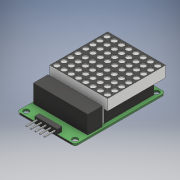
# Autodesk Inventor part: learnbotMatrizLed
Saved by Autodesk Inventor 2017 (Build 210142000, 142)
## iProperties
Part Number: learnbotMatrizLed
Material: Genérico
Document SubType Name: Modeling
Designer: rober
Density: 1 g/cm^3
Appearance: Valor por defecto
Author: rober
Autodesk Inventor part; units mm, degrees
ref_plane "YZ Plane" through (0, 0, 0) normal (1, 0, 0) x (0, 1, 0)
ref_plane "XZ Plane" through (0, 0, 0) normal (0, 1, 0) x (-1, 0, 0)
ref_plane "XY Plane" through (0, 0, 0) normal (0, 0, 1) x (1, 0, 0)
sketch "Boceto1" plane through (0, 0, 0) normal (0, 0, 1) x (1, 0, 0)
  line L0 (-0.15, 0.15) -> (-0.15, 4.85)
  line L1 (0, 5) -> (2.9, 5)
  line L2 (3.05, 4.85) -> (3.05, 0.15)
  line L3 (2.9, 0) -> (0, 0)
  arc A0 (2.9, 0) -> (3.05, 0.15) centre (2.9, 0.15) ccw
  arc A1 (-0.15, 0.15) -> (0, 0) centre (0, 0.15) ccw
  line L4 (3.05, 1.6) -> (3.05, 0.8)
  circle A2 centre (0.1, 0.25) radius 0.15
  circle A3 centre (2.8, 0.25) radius 0.15
  line L5 (0.925, 0) -> (0.925, -0.6)
  line L6 (0.975, 0) -> (0.975, -0.6)
  line L7 (0.925, -0.6) -> (0.975, -0.6)
  line L8 (1.175, 0) -> (1.175, -0.6)
  line L9 (1.225, 0) -> (1.225, -0.6)
  line L10 (1.175, -0.6) -> (1.225, -0.6)
  line L11 (1.425, 0) -> (1.425, -0.6)
  line L12 (1.475, 0) -> (1.475, -0.6)
  line L13 (1.425, -0.6) -> (1.475, -0.6)
  line L14 (1.675, 0) -> (1.675, -0.6)
  line L15 (1.725, 0) -> (1.725, -0.6)
  line L16 (1.675, -0.6) -> (1.725, -0.6)
  line L17 (1.925, 0) -> (1.925, -0.6)
  line L18 (1.975, 0) -> (1.975, -0.6)
  line L19 (1.925, -0.6) -> (1.975, -0.6)
  line L20 (0.925, 5) -> (0.925, 5.45)
  line L21 (0.975, 5) -> (0.975, 5.45)
  line L22 (0.925, 5.45) -> (0.975, 5.45)
  line L23 (1.175, 5) -> (1.175, 5.45)
  line L24 (1.225, 5) -> (1.225, 5.45)
  line L25 (1.175, 5.45) -> (1.225, 5.45)
  line L26 (1.425, 5) -> (1.425, 5.45)
  line L27 (1.475, 5) -> (1.475, 5.45)
  line L28 (1.425, 5.45) -> (1.475, 5.45)
  line L29 (1.675, 5) -> (1.675, 5.45)
  line L30 (1.725, 5) -> (1.725, 5.45)
  line L31 (1.675, 5.45) -> (1.725, 5.45)
  line L32 (1.925, 5) -> (1.925, 5.45)
  line L33 (1.975, 5) -> (1.975, 5.45)
  line L34 (1.925, 5.45) -> (1.975, 5.45)
  arc A4 (3.05, 4.85) -> (2.9, 5) centre (2.9, 4.85) ccw
  arc A5 (0, 5) -> (-0.15, 4.85) centre (0, 4.85) ccw
  circle A6 centre (0.1, 4.75) radius 0.15
  circle A7 centre (2.8, 4.75) radius 0.15
  constraints: 66 end point, 8 centre point, 8 point on circle, 2 point on line, 26 other
extrude "Extrusión1" add sketch "Boceto1" against normal blind 0.1 contours L0 A5 L1 A4 L2 A0 L3 A1
sketch "Boceto2" plane through (-0.15, 0.15, 0) normal (-1, 0, 0) x (0, 0, 1)
  line L0 (0.7, 4.85) -> (1.3, 4.85)
  line L1 (1.3, 4.85) -> (1.3, 1.65)
  line L2 (-0.1, 4.85) -> (-0.1, -0.15)
  line L3 (0, 1.65) -> (1.3, 1.65)
  line L4 (0, 1.45) -> (1, 1.45)
  line L5 (1, 1.45) -> (1, 0.65)
  line L6 (1, 0.65) -> (0, 0.65)
  line L7 (-0.1, -0.15) -> (0, -0.15)
  line L8 (0, -0.15) -> (0, 4.85)
  line L9 (0, 0.1) -> (0.25, 0.1)
  line L10 (0.25, 0.1) -> (0.25, -0.15)
  line L11 (0.25, -0.15) -> (0, -0.15)
  line L12 (0.1, -0.75) -> (0.15, -0.75)
  line L13 (0.15, -0.75) -> (0.15, -0.15)
  line L14 (0.1, -0.15) -> (0.1, -0.75)
  line L15 (0.1, 5.3) -> (0.15, 5.3)
  line L16 (0.15, 5.3) -> (0.15, 4.7)
  line L17 (0.1, 4.7) -> (0.1, 5.3)
  line L18 (1.3, 4.85) -> (0.7, 4.85)
  line L19 (0.7, 4.85) -> (0.7, 1.65)
  line L20 (0, 4.7) -> (0.7, 4.7)
  line L21 (0, 4.85) -> (-0.1, 4.85)
  constraints: 44 end point, 11 point on line
extrude "Extrusión2" add sketch "Boceto2" against normal blind 3.2 contours L0 L1 L3 L19 | L19 L3 L8 L20 | L4 L5 L6 L8
sketch "Boceto3" plane through (-0.15, 1.8, 1.3) normal (0, 0, 1) x (1, 0, 0)
  line L0 (0, -1.65) -> (0, 3.2)
  line L1 (0, 3.2) -> (3.2, 3.2)
  line L2 (3.2, 3.2) -> (3.2, -1.65)
  line L3 (3.05, -1.8) -> (0.15, -1.8)
  line L4 (3.2, 0) -> (0, 0)
  line L5 (3.2, -0.2) -> (3.2, -1)
  line L6 (3.2, -1) -> (0, -1)
  line L7 (3.2, -0.2) -> (0, -0.2)
  circle A0 centre (0.25, -1.55) radius 0.15
  circle A1 centre (2.95, -1.55) radius 0.15
  arc A2 (0, -1.65) -> (0.15, -1.8) centre (0.15, -1.65) ccw
  arc A3 (3.05, -1.8) -> (3.2, -1.65) centre (3.05, -1.65) ccw
  circle A4 centre (0.2, 0.1969) radius 0.15
  circle A5 centre (0.2, 0.5906) radius 0.15
  circle A6 centre (0.2, 0.9719) radius 0.15
  circle A7 centre (0.2, 1.3656) radius 0.15
  circle A8 centre (0.2, 1.7969) radius 0.15
  circle A9 centre (0.2, 2.1906) radius 0.15
  circle A10 centre (0.2, 2.5719) radius 0.15
  circle A11 centre (0.2, 2.9656) radius 0.15
  circle A12 centre (0.6, 0.1969) radius 0.15
  circle A13 centre (0.6, 0.5906) radius 0.15
  circle A14 centre (0.6, 0.9719) radius 0.15
  circle A15 centre (0.6, 1.3656) radius 0.15
  circle A16 centre (0.6, 1.7969) radius 0.15
  circle A17 centre (0.6, 2.1906) radius 0.15
  circle A18 centre (0.6, 2.5719) radius 0.15
  circle A19 centre (0.6, 2.9656) radius 0.15
  circle A20 centre (1, 0.1969) radius 0.15
  circle A21 centre (1, 0.5906) radius 0.15
  circle A22 centre (1, 0.9719) radius 0.15
  circle A23 centre (1, 1.3656) radius 0.15
  circle A24 centre (1, 1.7969) radius 0.15
  circle A25 centre (1, 2.1906) radius 0.15
  circle A26 centre (1, 2.5719) radius 0.15
  circle A27 centre (1, 2.9656) radius 0.15
  circle A28 centre (1.4, 0.1969) radius 0.15
  circle A29 centre (1.4, 0.5906) radius 0.15
  circle A30 centre (1.4, 0.9719) radius 0.15
  circle A31 centre (1.4, 1.3656) radius 0.15
  circle A32 centre (1.4, 1.7969) radius 0.15
  circle A33 centre (1.4, 2.1906) radius 0.15
  circle A34 centre (1.4, 2.5719) radius 0.15
  circle A35 centre (1.4, 2.9656) radius 0.15
  circle A36 centre (1.8, 0.1969) radius 0.15
  circle A37 centre (1.8, 0.5906) radius 0.15
  circle A38 centre (1.8, 0.9719) radius 0.15
  circle A39 centre (1.8, 1.3656) radius 0.15
  circle A40 centre (1.8, 1.7969) radius 0.15
  circle A41 centre (1.8, 2.1906) radius 0.15
  circle A42 centre (1.8, 2.5719) radius 0.15
  circle A43 centre (1.8, 2.9656) radius 0.15
  circle A44 centre (2.2, 0.1969) radius 0.15
  circle A45 centre (2.2, 0.5906) radius 0.15
  circle A46 centre (2.2, 0.9719) radius 0.15
  circle A47 centre (2.2, 1.3656) radius 0.15
  circle A48 centre (2.2, 1.7969) radius 0.15
  circle A49 centre (2.2, 2.1906) radius 0.15
  circle A50 centre (2.2, 2.5719) radius 0.15
  circle A51 centre (2.2, 2.9656) radius 0.15
  circle A52 centre (2.6, 0.1969) radius 0.15
  circle A53 centre (2.6, 0.5906) radius 0.15
  circle A54 centre (2.6, 0.9719) radius 0.15
  circle A55 centre (2.6, 1.3656) radius 0.15
  circle A56 centre (2.6, 1.7969) radius 0.15
  circle A57 centre (2.6, 2.1906) radius 0.15
  circle A58 centre (2.6, 2.5719) radius 0.15
  circle A59 centre (2.6, 2.9656) radius 0.15
  circle A60 centre (3, 0.1969) radius 0.15
  circle A61 centre (3, 0.5906) radius 0.15
  circle A62 centre (3, 0.9719) radius 0.15
  circle A63 centre (3, 1.3656) radius 0.15
  circle A64 centre (3, 1.7969) radius 0.15
  circle A65 centre (3, 2.1906) radius 0.15
  circle A66 centre (3, 2.5719) radius 0.15
  circle A67 centre (3, 2.9656) radius 0.15
  line L8 (0.975, -1.8) -> (0.975, -1.55)
  line L9 (0.975, -1.55) -> (2.225, -1.55)
  line L10 (2.225, -1.55) -> (2.225, -1.8)
  line L11 (1.225, -1.8) -> (1.225, -1.55)
  line L12 (1.475, -1.8) -> (1.475, -1.55)
  line L13 (1.725, -1.8) -> (1.725, -1.55)
  line L14 (1.975, -1.8) -> (1.975, -1.55)
  line L15 (1.075, -1.8) -> (1.075, -2.4)
  line L16 (1.125, -1.8) -> (1.125, -2.4)
  line L17 (1.075, -2.4) -> (1.125, -2.4)
  line L18 (1.325, -1.8) -> (1.325, -2.4)
  line L19 (1.375, -1.8) -> (1.375, -2.4)
  line L20 (1.325, -2.4) -> (1.375, -2.4)
  line L21 (1.575, -1.8) -> (1.575, -2.4)
  line L22 (1.625, -1.8) -> (1.625, -2.4)
  line L23 (1.575, -2.4) -> (1.625, -2.4)
  line L24 (1.825, -1.8) -> (1.825, -2.4)
  line L25 (1.875, -1.8) -> (1.875, -2.4)
  line L26 (1.825, -2.4) -> (1.875, -2.4)
  line L27 (2.075, -1.8) -> (2.075, -2.4)
  line L28 (2.125, -1.8) -> (2.125, -2.4)
  line L29 (2.075, -2.4) -> (2.125, -2.4)
  line L30 (1.075, 3.2) -> (1.075, 3.65)
  line L31 (1.125, 3.2) -> (1.125, 3.65)
  line L32 (1.075, 3.65) -> (1.125, 3.65)
  line L33 (1.325, 3.2) -> (1.325, 3.65)
  line L34 (1.375, 3.2) -> (1.375, 3.65)
  line L35 (1.325, 3.65) -> (1.375, 3.65)
  line L36 (1.575, 3.2) -> (1.575, 3.65)
  line L37 (1.625, 3.2) -> (1.625, 3.65)
  line L38 (1.575, 3.65) -> (1.625, 3.65)
  line L39 (1.825, 3.2) -> (1.825, 3.65)
  line L40 (1.875, 3.2) -> (1.875, 3.65)
  line L41 (1.825, 3.65) -> (1.875, 3.65)
  line L42 (2.075, 3.2) -> (2.075, 3.65)
  line L43 (2.125, 3.2) -> (2.125, 3.65)
  line L44 (2.075, 3.65) -> (2.125, 3.65)
  line L45 (0, 0) -> (0, 3.2) projected
  line L46 (0, 0) -> (3.2, 0) projected
  line L47 (3.2, 3.2) -> (3.2, 0) projected
  line L48 (0, 3.2) -> (3.2, 3.2) projected
  point P0 (0.15, -1.8)
  constraints: 86 end point, 68 centre point, 10 point on line, 4 point on circle, 32 other
extrude "Extrusión3" cut sketch "Boceto3" against normal blind 0.05 contours A4 | A5 | A6 | A7 | A8 | A9 | A10 | A11 | A12 | A13 | A14 | A15 | A16 | A17 | A18 | A19 | A20 | A21 | A22 | A23 | A24 | A25 | A26 | A27 | A28 | A29 | A30 | A31 | A32 | A33 | A34 | A35 | A36 | A37 | A38 | A39 | A40 | A41 | A42 | A43 | A44 | A45 | A46 | A47 | A48 | A49 | A50 | A51 | A52 | A53 | A54 | A55 | A56 | A57 | A58 | A59 | A60 | A61 | A62 | A63 | A64 | A65 | A66 | A67
sketch "Boceto4" plane through (0, 0, 0) normal (0, 0, 1) x (1, 0, 0)
  line L0 (-0.15, 0.15) -> (-0.15, 5)
  line L1 (-0.15, 5) -> (3.05, 5)
  line L2 (3.05, 5) -> (3.05, 0.15)
  line L3 (2.9, 0) -> (0, 0)
  line L4 (3.05, 1.8) -> (-0.15, 1.8)
  line L5 (3.05, 1.6) -> (3.05, 0.8)
  line L6 (3.05, 0.8) -> (-0.15, 0.8)
  line L7 (3.05, 1.6) -> (-0.15, 1.6)
  circle A0 centre (0.1, 0.25) radius 0.15
  circle A1 centre (2.8, 0.25) radius 0.15
  arc A2 (-0.15, 0.15) -> (0, 0) centre (0, 0.15) ccw
  arc A3 (2.9, 0) -> (3.05, 0.15) centre (2.9, 0.15) ccw
  circle A4 centre (0.05, 1.9969) radius 0.15
  circle A5 centre (0.05, 2.3906) radius 0.15
  circle A6 centre (0.05, 2.7719) radius 0.15
  circle A7 centre (0.05, 3.1656) radius 0.15
  circle A8 centre (0.05, 3.5969) radius 0.15
  circle A9 centre (0.05, 3.9906) radius 0.15
  circle A10 centre (0.05, 4.3719) radius 0.15
  circle A11 centre (0.05, 4.7656) radius 0.15
  circle A12 centre (0.45, 1.9969) radius 0.15
  circle A13 centre (0.45, 2.3906) radius 0.15
  circle A14 centre (0.45, 2.7719) radius 0.15
  circle A15 centre (0.45, 3.1656) radius 0.15
  circle A16 centre (0.45, 3.5969) radius 0.15
  circle A17 centre (0.45, 3.9906) radius 0.15
  circle A18 centre (0.45, 4.3719) radius 0.15
  circle A19 centre (0.45, 4.7656) radius 0.15
  circle A20 centre (0.85, 1.9969) radius 0.15
  circle A21 centre (0.85, 2.3906) radius 0.15
  circle A22 centre (0.85, 2.7719) radius 0.15
  circle A23 centre (0.85, 3.1656) radius 0.15
  circle A24 centre (0.85, 3.5969) radius 0.15
  circle A25 centre (0.85, 3.9906) radius 0.15
  circle A26 centre (0.85, 4.3719) radius 0.15
  circle A27 centre (0.85, 4.7656) radius 0.15
  circle A28 centre (1.25, 1.9969) radius 0.15
  circle A29 centre (1.25, 2.3906) radius 0.15
  circle A30 centre (1.25, 2.7719) radius 0.15
  circle A31 centre (1.25, 3.1656) radius 0.15
  circle A32 centre (1.25, 3.5969) radius 0.15
  circle A33 centre (1.25, 3.9906) radius 0.15
  circle A34 centre (1.25, 4.3719) radius 0.15
  circle A35 centre (1.25, 4.7656) radius 0.15
  circle A36 centre (1.65, 1.9969) radius 0.15
  circle A37 centre (1.65, 2.3906) radius 0.15
  circle A38 centre (1.65, 2.7719) radius 0.15
  circle A39 centre (1.65, 3.1656) radius 0.15
  circle A40 centre (1.65, 3.5969) radius 0.15
  circle A41 centre (1.65, 3.9906) radius 0.15
  circle A42 centre (1.65, 4.3719) radius 0.15
  circle A43 centre (1.65, 4.7656) radius 0.15
  circle A44 centre (2.05, 1.9969) radius 0.15
  circle A45 centre (2.05, 2.3906) radius 0.15
  circle A46 centre (2.05, 2.7719) radius 0.15
  circle A47 centre (2.05, 3.1656) radius 0.15
  circle A48 centre (2.05, 3.5969) radius 0.15
  circle A49 centre (2.05, 3.9906) radius 0.15
  circle A50 centre (2.05, 4.3719) radius 0.15
  circle A51 centre (2.05, 4.7656) radius 0.15
  circle A52 centre (2.45, 1.9969) radius 0.15
  circle A53 centre (2.45, 2.3906) radius 0.15
  circle A54 centre (2.45, 2.7719) radius 0.15
  circle A55 centre (2.45, 3.1656) radius 0.15
  circle A56 centre (2.45, 3.5969) radius 0.15
  circle A57 centre (2.45, 3.9906) radius 0.15
  circle A58 centre (2.45, 4.3719) radius 0.15
  circle A59 centre (2.45, 4.7656) radius 0.15
  circle A60 centre (2.85, 1.9969) radius 0.15
  circle A61 centre (2.85, 2.3906) radius 0.15
  circle A62 centre (2.85, 2.7719) radius 0.15
  circle A63 centre (2.85, 3.1656) radius 0.15
  circle A64 centre (2.85, 3.5969) radius 0.15
  circle A65 centre (2.85, 3.9906) radius 0.15
  circle A66 centre (2.85, 4.3719) radius 0.15
  circle A67 centre (2.85, 4.7656) radius 0.15
  line L8 (0.825, 0) -> (0.825, 0.25)
  line L9 (0.825, 0.25) -> (2.075, 0.25)
  line L10 (2.075, 0.25) -> (2.075, 0)
  line L11 (1.075, 0) -> (1.075, 0.25)
  line L12 (1.325, 0) -> (1.325, 0.25)
  line L13 (1.575, 0) -> (1.575, 0.25)
  line L14 (1.825, 0) -> (1.825, 0.25)
  line L15 (0.925, 0) -> (0.925, -0.6)
  line L16 (0.975, 0) -> (0.975, -0.6)
  line L17 (0.925, -0.6) -> (0.975, -0.6)
  line L18 (1.175, 0) -> (1.175, -0.6)
  line L19 (1.225, 0) -> (1.225, -0.6)
  line L20 (1.175, -0.6) -> (1.225, -0.6)
  line L21 (1.425, 0) -> (1.425, -0.6)
  line L22 (1.475, 0) -> (1.475, -0.6)
  line L23 (1.425, -0.6) -> (1.475, -0.6)
  line L24 (1.675, 0) -> (1.675, -0.6)
  line L25 (1.725, 0) -> (1.725, -0.6)
  line L26 (1.675, -0.6) -> (1.725, -0.6)
  line L27 (1.925, 0) -> (1.925, -0.6)
  line L28 (1.975, 0) -> (1.975, -0.6)
  line L29 (1.925, -0.6) -> (1.975, -0.6)
  line L30 (0.925, 5) -> (0.925, 5.45)
  line L31 (0.975, 5) -> (0.975, 5.45)
  line L32 (0.925, 5.45) -> (0.975, 5.45)
  line L33 (1.175, 5) -> (1.175, 5.45)
  line L34 (1.225, 5) -> (1.225, 5.45)
  line L35 (1.175, 5.45) -> (1.225, 5.45)
  line L36 (1.425, 5) -> (1.425, 5.45)
  line L37 (1.475, 5) -> (1.475, 5.45)
  line L38 (1.425, 5.45) -> (1.475, 5.45)
  line L39 (1.675, 5) -> (1.675, 5.45)
  line L40 (1.725, 5) -> (1.725, 5.45)
  line L41 (1.675, 5.45) -> (1.725, 5.45)
  line L42 (1.925, 5) -> (1.925, 5.45)
  line L43 (1.975, 5) -> (1.975, 5.45)
  line L44 (1.925, 5.45) -> (1.975, 5.45)
  circle A68 centre (0.1, 0.25) radius 0.15 projected
  point P0 (0, 0)
  constraints: 86 end point, 68 centre point, 10 point on line, 4 point on circle, 32 other
extrude "Extrusión4" add sketch "Boceto4" along normal blind 0.25 contours L8 L9 L11 L3 | L9 L12 L3 L11 | L3 L14 L9 L10 | L9 L13 L3 L12 | L9 L14 L3 L13
sketch "Boceto5" plane through (0, 0, -0.1) normal (0, -1, 0) x (1, 0, 0)
  line L0 (0.825, 0.35) -> (2.075, 0.35) projected
  line L1 (0.825, 0.35) -> (1.075, 0.35)
  line L2 (1.075, 0.35) -> (1.075, 0.1)
  line L3 (3.05, 0.1) -> (-0.15, 0.1) projected
  line L4 (0.825, 0.1) -> (0.825, 0.35) projected
  line L5 (0.975, 0.25) -> (0.975, 0.2)
  line L6 (0.975, 0.2) -> (0.925, 0.2)
  line L7 (0.925, 0.2) -> (0.925, 0.25)
  line L8 (0.925, 0.25) -> (0.975, 0.25)
  line L9 (1.325, 0.35) -> (1.325, 0.1)
  line L10 (1.225, 0.25) -> (1.225, 0.2)
  line L11 (1.225, 0.2) -> (1.175, 0.2)
  line L12 (1.175, 0.2) -> (1.175, 0.25)
  line L13 (1.175, 0.25) -> (1.225, 0.25)
  line L14 (1.575, 0.35) -> (1.575, 0.1)
  line L15 (1.475, 0.25) -> (1.475, 0.2)
  line L16 (1.475, 0.2) -> (1.425, 0.2)
  line L17 (1.425, 0.2) -> (1.425, 0.25)
  line L18 (1.425, 0.25) -> (1.475, 0.25)
  line L19 (1.825, 0.35) -> (1.825, 0.1)
  line L20 (1.725, 0.25) -> (1.725, 0.2)
  line L21 (1.725, 0.2) -> (1.675, 0.2)
  line L22 (1.675, 0.2) -> (1.675, 0.25)
  line L23 (1.675, 0.25) -> (1.725, 0.25)
  line L24 (2.075, 0.35) -> (2.075, 0.1)
  line L25 (1.975, 0.25) -> (1.975, 0.2)
  line L26 (1.975, 0.2) -> (1.925, 0.2)
  line L27 (1.925, 0.2) -> (1.925, 0.25)
  line L28 (1.925, 0.25) -> (1.975, 0.25)
  point P0 (0, 0.1)
  dimension "d8" = 0.25
  dimension "d9" = 0.25
  dimension "d15" = 0.25
  dimension "d16" = 0.25
  dimension "d17" = 0.25
  dimension "d18" = 0.25
  constraints: 52 end point, 5 horizontal, 2 point on line, 1 perpendicular
  measures "d8" distance of L0.start L1.end
  measures "d9" distance of L1.end L2.end
  measures "d15" distance of L9.start L9.end
  measures "d16" distance of L14.start L14.end
  measures "d17" distance of L19.start L19.end
  measures "d18" distance of L24.start L24.end
extrude "Extrusión5" add sketch "Boceto5" along normal blind 0.6 contours L5 L6 L7 L8 | L10 L11 L12 L13 | L15 L16 L17 L18 | L20 L21 L22 L23 | L25 L26 L27 L28
sketch "Boceto6" plane through (0, 0, 0) normal (0, 0, 1) x (1, 0, 0)
  line L0 (3.05, 4.85) -> (3.05, 0)
  line L1 (3.05, 0) -> (-0.15, 0)
  line L2 (-0.15, 0) -> (-0.15, 4.85)
  line L3 (0, 4.85) -> (2.9, 4.85)
  line L4 (-0.15, 3.2) -> (3.05, 3.2)
  line L5 (-0.15, 3.4) -> (-0.15, 4.2)
  line L6 (-0.15, 4.2) -> (3.05, 4.2)
  line L7 (-0.15, 3.4) -> (3.05, 3.4)
  circle A0 centre (2.8, 4.75) radius 0.15
  circle A1 centre (0.1, 4.75) radius 0.15
  arc A2 (3.05, 4.85) -> (2.9, 5) centre (2.9, 4.85) ccw
  arc A3 (0, 5) -> (-0.15, 4.85) centre (0, 4.85) ccw
  circle A4 centre (2.85, 3.0031) radius 0.15
  circle A5 centre (2.85, 2.6094) radius 0.15
  circle A6 centre (2.85, 2.2281) radius 0.15
  circle A7 centre (2.85, 1.8344) radius 0.15
  circle A8 centre (2.85, 1.4031) radius 0.15
  circle A9 centre (2.85, 1.0094) radius 0.15
  circle A10 centre (2.85, 0.6281) radius 0.15
  circle A11 centre (2.85, 0.2344) radius 0.15
  circle A12 centre (2.45, 3.0031) radius 0.15
  circle A13 centre (2.45, 2.6094) radius 0.15
  circle A14 centre (2.45, 2.2281) radius 0.15
  circle A15 centre (2.45, 1.8344) radius 0.15
  circle A16 centre (2.45, 1.4031) radius 0.15
  circle A17 centre (2.45, 1.0094) radius 0.15
  circle A18 centre (2.45, 0.6281) radius 0.15
  circle A19 centre (2.45, 0.2344) radius 0.15
  circle A20 centre (2.05, 3.0031) radius 0.15
  circle A21 centre (2.05, 2.6094) radius 0.15
  circle A22 centre (2.05, 2.2281) radius 0.15
  circle A23 centre (2.05, 1.8344) radius 0.15
  circle A24 centre (2.05, 1.4031) radius 0.15
  circle A25 centre (2.05, 1.0094) radius 0.15
  circle A26 centre (2.05, 0.6281) radius 0.15
  circle A27 centre (2.05, 0.2344) radius 0.15
  circle A28 centre (1.65, 3.0031) radius 0.15
  circle A29 centre (1.65, 2.6094) radius 0.15
  circle A30 centre (1.65, 2.2281) radius 0.15
  circle A31 centre (1.65, 1.8344) radius 0.15
  circle A32 centre (1.65, 1.4031) radius 0.15
  circle A33 centre (1.65, 1.0094) radius 0.15
  circle A34 centre (1.65, 0.6281) radius 0.15
  circle A35 centre (1.65, 0.2344) radius 0.15
  circle A36 centre (1.25, 3.0031) radius 0.15
  circle A37 centre (1.25, 2.6094) radius 0.15
  circle A38 centre (1.25, 2.2281) radius 0.15
  circle A39 centre (1.25, 1.8344) radius 0.15
  circle A40 centre (1.25, 1.4031) radius 0.15
  circle A41 centre (1.25, 1.0094) radius 0.15
  circle A42 centre (1.25, 0.6281) radius 0.15
  circle A43 centre (1.25, 0.2344) radius 0.15
  circle A44 centre (0.85, 3.0031) radius 0.15
  circle A45 centre (0.85, 2.6094) radius 0.15
  circle A46 centre (0.85, 2.2281) radius 0.15
  circle A47 centre (0.85, 1.8344) radius 0.15
  circle A48 centre (0.85, 1.4031) radius 0.15
  circle A49 centre (0.85, 1.0094) radius 0.15
  circle A50 centre (0.85, 0.6281) radius 0.15
  circle A51 centre (0.85, 0.2344) radius 0.15
  circle A52 centre (0.45, 3.0031) radius 0.15
  circle A53 centre (0.45, 2.6094) radius 0.15
  circle A54 centre (0.45, 2.2281) radius 0.15
  circle A55 centre (0.45, 1.8344) radius 0.15
  circle A56 centre (0.45, 1.4031) radius 0.15
  circle A57 centre (0.45, 1.0094) radius 0.15
  circle A58 centre (0.45, 0.6281) radius 0.15
  circle A59 centre (0.45, 0.2344) radius 0.15
  circle A60 centre (0.05, 3.0031) radius 0.15
  circle A61 centre (0.05, 2.6094) radius 0.15
  circle A62 centre (0.05, 2.2281) radius 0.15
  circle A63 centre (0.05, 1.8344) radius 0.15
  circle A64 centre (0.05, 1.4031) radius 0.15
  circle A65 centre (0.05, 1.0094) radius 0.15
  circle A66 centre (0.05, 0.6281) radius 0.15
  circle A67 centre (0.05, 0.2344) radius 0.15
  line L8 (2.075, 4.85) -> (2.075, 4.6)
  line L9 (2.075, 4.6) -> (0.825, 4.6)
  line L10 (0.825, 4.6) -> (0.825, 4.85)
  line L11 (1.825, 4.85) -> (1.825, 4.6)
  line L12 (1.575, 4.85) -> (1.575, 4.6)
  line L13 (1.325, 4.85) -> (1.325, 4.6)
  line L14 (1.075, 4.85) -> (1.075, 4.6)
  line L15 (1.975, 4.85) -> (1.975, 5.45)
  line L16 (1.925, 4.85) -> (1.925, 5.45)
  line L17 (1.975, 5.45) -> (1.925, 5.45)
  line L18 (1.725, 4.85) -> (1.725, 5.45)
  line L19 (1.675, 4.85) -> (1.675, 5.45)
  line L20 (1.725, 5.45) -> (1.675, 5.45)
  line L21 (1.475, 4.85) -> (1.475, 5.45)
  line L22 (1.425, 4.85) -> (1.425, 5.45)
  line L23 (1.475, 5.45) -> (1.425, 5.45)
  line L24 (1.225, 4.85) -> (1.225, 5.45)
  line L25 (1.175, 4.85) -> (1.175, 5.45)
  line L26 (1.225, 5.45) -> (1.175, 5.45)
  line L27 (0.975, 4.85) -> (0.975, 5.45)
  line L28 (0.925, 4.85) -> (0.925, 5.45)
  line L29 (0.975, 5.45) -> (0.925, 5.45)
  line L30 (1.975, 0) -> (1.975, -0.45)
  line L31 (1.925, 0) -> (1.925, -0.45)
  line L32 (1.975, -0.45) -> (1.925, -0.45)
  line L33 (1.725, 0) -> (1.725, -0.45)
  line L34 (1.675, 0) -> (1.675, -0.45)
  line L35 (1.725, -0.45) -> (1.675, -0.45)
  line L36 (1.475, 0) -> (1.475, -0.45)
  line L37 (1.425, 0) -> (1.425, -0.45)
  line L38 (1.475, -0.45) -> (1.425, -0.45)
  line L39 (1.225, 0) -> (1.225, -0.45)
  line L40 (1.175, 0) -> (1.175, -0.45)
  line L41 (1.225, -0.45) -> (1.175, -0.45)
  line L42 (0.975, 0) -> (0.975, -0.45)
  line L43 (0.925, 0) -> (0.925, -0.45)
  line L44 (0.975, -0.45) -> (0.925, -0.45)
  circle A68 centre (2.8, 4.75) radius 0.15 projected
  line L45 (0.825, 4.6) -> (0.825, 4.45)
  point P0 (0, 0)
  constraints: 88 end point, 68 centre point, 10 point on line, 4 point on circle, 1 vertical, 32 other
sketch "Boceto7" plane through (-0.15, 4.85, 0.7) normal (0, 1, 0) x (1, 0, 0)
  line L0 (0, 0) -> (0, 0.7) projected
  line L1 (3.2, 0) -> (0, 0) projected
  line L2 (3.2, 0.7) -> (3.2, 0) projected
  line L3 (3.0618, 0.7) -> (3.2, 0.7) projected
  line L4 (2.8382, 0.7) -> (3.0618, 0.7) projected
  line L5 (0.3618, 0.7) -> (2.8382, 0.7) projected
  line L6 (0.1382, 0.7) -> (0.3618, 0.7) projected
  line L7 (0, 0.7) -> (0.1382, 0.7) projected
  point P0 (0.15, 0.7)
extrude "Extrusión6" cut sketch "Boceto7" against normal blind 0.3
extrude "Extrusión7" add sketch "Boceto6" along normal blind 0.25 contours L3 L14 L9 L10 | L14 L3 L13 L9 | L13 L3 L12 L9 | L12 L3 L11 L9 | L11 L3 L8 L9
sketch "Boceto8" plane through (0.825, 4.85, 0) normal (0, 1, 0) x (1, 0, 0)
  line L0 (0, 0) -> (1.25, 0) projected
  line L1 (0, 0) -> (0, -0.25) projected
  line L2 (1.25, -0.25) -> (0, -0.25) projected
  line L3 (1.25, 0) -> (1.25, -0.25) projected
  line L4 (1.25, -0.25) -> (1, -0.25)
  line L5 (1.25, -0.25) -> (0, -0.25) projected
  line L6 (1, -0.25) -> (1, 0)
  line L7 (2.075, 0) -> (-0.825, 0) projected
  line L8 (1.125, -0.15) -> (1.1, -0.15)
  line L9 (1.1, -0.15) -> (1.1, -0.1)
  line L10 (1.1, -0.1) -> (1.15, -0.1)
  line L11 (1.15, -0.1) -> (1.15, -0.15)
  line L12 (1.15, -0.15) -> (1.125, -0.15)
  line L13 (0.75, -0.25) -> (0.75, 0)
  line L14 (0.875, -0.15) -> (0.85, -0.15)
  line L15 (0.85, -0.15) -> (0.85, -0.1)
  line L16 (0.85, -0.1) -> (0.9, -0.1)
  line L17 (0.9, -0.1) -> (0.9, -0.15)
  line L18 (0.9, -0.15) -> (0.875, -0.15)
  line L19 (0.5, -0.25) -> (0.5, 0)
  line L20 (0.625, -0.15) -> (0.6, -0.15)
  line L21 (0.6, -0.15) -> (0.6, -0.1)
  line L22 (0.6, -0.1) -> (0.65, -0.1)
  line L23 (0.65, -0.1) -> (0.65, -0.15)
  line L24 (0.65, -0.15) -> (0.625, -0.15)
  line L25 (0.25, -0.25) -> (0.25, 0)
  line L26 (0.375, -0.15) -> (0.35, -0.15)
  line L27 (0.35, -0.15) -> (0.35, -0.1)
  line L28 (0.35, -0.1) -> (0.4, -0.1)
  line L29 (0.4, -0.1) -> (0.4, -0.15)
  line L30 (0.4, -0.15) -> (0.375, -0.15)
  line L31 (0, -0.25) -> (0, 0)
  line L32 (0.125, -0.15) -> (0.1, -0.15)
  line L33 (0.1, -0.15) -> (0.1, -0.1)
  line L34 (0.1, -0.1) -> (0.15, -0.1)
  line L35 (0.15, -0.1) -> (0.15, -0.15)
  line L36 (0.15, -0.15) -> (0.125, -0.15)
  dimension "d26" = 0.25
  constraints: 62 end point, 6 perpendicular, 2 point on line
  measures "d26" distance of L2.start L4.end
extrude "Extrusión8" add sketch "Boceto8" along normal blind 0.6 contours L14 L15 L16 L17 L18 | L20 L21 L22 L23 L24 | L26 L27 L28 L29 L30 | L32 L33 L34 L35 L36
sketch "Boceto9" plane through (-0.15, 0.15, -0.1) normal (-1, 0, 0) x (0, 0, 1)
  line L0 (0.8, 4.4) -> (0.8, 4.85) projected
  line L1 (0.8, 4.4) -> (0.8, 1.65)
  line L2 (0.1, 1.65) -> (1.4, 1.65) projected
  line L3 (0.1, 1.65) -> (0.8, 1.65)
  line L4 (0.8, 1.65) -> (0.8, 4.4)
  line L5 (0.8, 4.4) -> (0.1, 4.4)
  line L6 (0.1, 4.4) -> (0.1, 1.65)
  point P0 (0.1, -0.15)
  constraints: 10 end point, 2 parallel, 1 horizontal, 1 perpendicular, 1 point on line, 1 vertical
extrude "Extrusión9" cut sketch "Boceto9" against normal blind 0.2
sketch "Boceto10" plane through (3.05, 0.15, -0.1) normal (1, 0, 0) x (0, 0, -1)
  line L0 (-0.1, 4.4) -> (-0.8, 4.4) projected
  line L1 (-0.1, 4.4) -> (-0.8, 4.4) projected
  line L2 (-0.8, 1.65) -> (-1.4, 1.65) projected
  line L3 (-0.8, 4.4) -> (-0.8, 1.65)
  line L4 (-0.1, 4.4) -> (-0.8, 4.4)
  line L5 (-0.8, 4.4) -> (-0.8, 1.65)
  line L6 (-0.8, 1.65) -> (-0.1, 1.65)
  line L7 (-0.1, 1.65) -> (-0.1, 4.4)
  point P0 (-0.1, -0.15)
  constraints: 10 end point, 2 parallel, 1 horizontal, 1 perpendicular, 1 vertical
extrude "Extrusión10" cut sketch "Boceto10" against normal blind 0.2
sketch "Boceto11" plane through (-0.15, 0.15, -0.1) normal (-1, 0, 0) x (0, 0, 1)
  line L0 (1.1, 0.65) -> (1.1, 1.45) projected
  line L1 (0.1, 0.65) -> (1.1, 0.65) projected
  line L2 (1.1, 0.65) -> (0.1, 0.65) projected
  line L3 (1.1, 1.45) -> (0.1, 1.45)
  line L4 (0.1, 1.45) -> (0.1, 0.65)
  line L5 (0.1, 0.65) -> (1.1, 0.65)
  line L6 (1.1, 0.65) -> (1.1, 1.45)
  point P0 (0.1, -0.15)
  constraints: 8 end point, 2 parallel, 1 horizontal, 1 perpendicular
extrude "Extrusión11" cut sketch "Boceto11" against normal blind 0.1
sketch "Boceto12" plane through (3.05, 0.15, -0.1) normal (1, 0, 0) x (0, 0, -1)
  line L0 (-1.1, 1.45) -> (-1.1, 0.65) projected
  line L1 (-0.1, 1.45) -> (-1.1, 1.45) projected
  line L2 (-1.1, 0.65) -> (-0.1, 0.65)
  line L3 (-0.1, 0.65) -> (-0.1, 1.45)
  line L4 (-0.1, 1.45) -> (-1.1, 1.45)
  line L5 (-1.1, 1.45) -> (-1.1, 0.65)
  point P0 (-0.1, -0.15)
  constraints: 8 end point, 2 parallel, 1 horizontal, 1 perpendicular
extrude "Extrusión12" cut sketch "Boceto12" against normal blind 0.1
